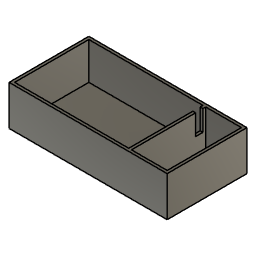
Board Case v2 (Autodesk Fusion 360 design; units mm, degrees)
Autodesk Fusion 360 part; units mm, degrees
sketch "Sketch1" plane through (0, 0, 0) normal (0, 0, 1) x (1, 0, 0)
  line L0 (57.5, -29) -> (-57.5, -29)
  line L1 (-57.5, -29) -> (-57.5, 29)
  line L2 (-57.5, 29) -> (57.5, 29)
  line L3 (57.5, 29) -> (57.5, -29)
  line L4 (57.5, -29) -> (-57.5, 29) construction
  line L5 (-57.5, -29) -> (57.5, 29) construction
  line L6 (55.5, -27) -> (-55.5, -27)
  line L7 (-55.5, -27) -> (-55.5, 27)
  line L8 (-55.5, 27) -> (55.5, 27)
  line L9 (55.5, 27) -> (55.5, -27)
  line L10 (55.5, -27) -> (-55.5, 27) construction
  line L11 (-55.5, -27) -> (55.5, 27) construction
  constraint horizontal L0
  constraint perpendicular L0 L1
  constraint parallel L0 L2
  constraint parallel L1 L3
  constraint coincident L4 origin
  constraint coincident L5 origin
  constraint horizontal L6
  constraint perpendicular L6 L7
  constraint parallel L6 L8
  constraint parallel L7 L9
  constraint coincident L10 origin
  constraint coincident L11 origin
extrude "Extrude1" add sketch "Sketch1" along normal blind 2 contours L0 L1 L2 L3 | L6 L7 L8 L9
sketch "Sketch2" plane through (0, 0, 2) normal (0, 0, 1) x (-1, 0, 0)
  line L0 (-57.5, -29) -> (57.5, -29)
  line L1 (57.5, -29) -> (57.5, 29)
  line L2 (57.5, 29) -> (-57.5, 29)
  line L3 (-57.5, 29) -> (-57.5, -29)
  line L4 (-57.5, 29) -> (57.5, 29)
  line L5 (57.5, 29) -> (57.5, -29)
  line L6 (57.5, -29) -> (-57.5, -29)
  line L7 (-57.5, -29) -> (-57.5, 29)
  line L8 (-57.5, 29) -> (57.5, -29) construction
  line L9 (57.5, 29) -> (-57.5, -29) construction
  line L10 (-55.5, 27) -> (55.5, 27)
  line L11 (55.5, 27) -> (55.5, -27)
  line L12 (55.5, -27) -> (-55.5, -27)
  line L13 (-55.5, -27) -> (-55.5, 27)
  line L14 (-55.5, 27) -> (55.5, -27) construction
  line L15 (55.5, 27) -> (-55.5, -27) construction
  constraint horizontal L4
  constraint perpendicular L4 L5
  constraint parallel L4 L6
  constraint parallel L5 L7
  constraint coincident L8 origin
  constraint coincident L9 origin
  constraint coincident L2.end L3.start
  constraint horizontal L10
  constraint perpendicular L10 L11
  constraint parallel L10 L12
  constraint parallel L11 L13
  constraint coincident L14 origin
  constraint coincident L15 origin
extrude "Extrude2" add sketch "Sketch2" along normal blind 27
sketch "Sketch3" plane through (0, 0, 2) normal (0, 0, 1) x (-1, 0, 0)
  line L0 (55.5, -27) -> (55.5, 27)
  line L1 (55.5, 27) -> (-55.5, 27)
  line L2 (-55.5, 27) -> (-55.5, -27)
  line L3 (-55.5, -27) -> (55.5, -27)
  line L4 (-55.5, -27) -> (-29.5, -27)
  line L5 (-29.5, -27) -> (-29.5, 27)
  line L6 (-29.5, 27) -> (-55.5, 27)
  line L7 (-55.5, 27) -> (-55.5, -27)
  line L8 (-29.5, -27) -> (-27.5, -27)
  line L9 (-27.5, -27) -> (-27.5, 27)
  line L10 (-27.5, 27) -> (-29.5, 27)
  line L11 (-29.5, 27) -> (-29.5, -27)
  constraint horizontal L4
  constraint vertical L5
  constraint horizontal L6
  constraint vertical L7
  constraint coincident L2.end L3.start
  constraint horizontal L8
  constraint vertical L9
  constraint horizontal L10
  constraint vertical L11
extrude "Extrude3" add sketch "Sketch3" along normal blind 27 contours L1 L3 L5 L8 L9 L10 L11
sketch "Sketch4" plane through (0, 0, 29) normal (0, 0, 1) x (-1, 0, 0)
  line L0 (-27.5, 27) -> (55.5, 27)
  line L1 (55.5, 27) -> (55.5, -27)
  line L2 (55.5, -27) -> (-27.5, -27)
  line L3 (-27.5, -27) -> (-27.5, 27)
  line L4 (-29.5, 27) -> (-29.5, -27)
  line L5 (-29.5, -27) -> (-55.5, -27)
  line L6 (-55.5, -27) -> (-55.5, 27)
  line L7 (-55.5, 27) -> (-29.5, 27)
  line L8 (-57.5, -29) -> (57.5, -29)
  line L9 (57.5, -29) -> (57.5, 29)
  line L10 (57.5, 29) -> (-57.5, 29)
  line L11 (-57.5, 29) -> (-57.5, -29)
  line L12 (-25, -25) -> (-32.1654, -25)
  line L13 (-32.1654, -25) -> (-32.1654, -19.6955)
  line L14 (-32.1654, -19.6955) -> (-25, -19.6955)
  line L15 (-25, -19.6955) -> (-25, -25)
  constraint horizontal L12
  constraint vertical L13
  constraint horizontal L14
  constraint vertical L15
extrude "Extrude4" cut sketch "Sketch4" against normal blind 15 contours L3 L12 L14 L15 | L3 L4 L12 L14 | L4 L12 L13 L14
